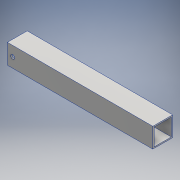
# Autodesk Inventor part: front_arm_rect
Saved by Autodesk Inventor 2016 (Build 200138000, 138)
## iProperties
Created: 2016-09-24
Part Number: front_arm_rect
Material: Aluminum 6061
Document SubType Name: Modeling
Designer: Jakub
Density: 2.7 g/cm^3
Appearance: Aluminum - Flat
Author: Jakub
Autodesk Inventor part; units mm, degrees
ref_plane "YZ Plane" through (0, 0, 0) normal (1, 0, 0) x (0, 1, 0)
ref_plane "XZ Plane" through (0, 0, 0) normal (0, 1, 0) x (-1, 0, 0)
ref_plane "XY Plane" through (0, 0, 0) normal (0, 0, 1) x (1, 0, 0)
sketch "Sketch1" plane through (0, 0, 0) normal (1, 0, 0) x (0, 1, 0)
  line L0 (-7.5, 7.5) -> (7.5, 7.5)
  line L1 (7.5, 7.5) -> (7.5, -7.5)
  line L2 (7.5, -7.5) -> (-7.5, -7.5)
  line L3 (-7.5, -7.5) -> (-7.5, 7.5)
  line L4 (-7.5, 7.5) -> (7.5, -7.5) construction
  line L5 (7.5, 7.5) -> (-7.5, -7.5) construction
  line L6 (-6.5, 6.5) -> (6.5, 6.5)
  line L7 (6.5, 6.5) -> (6.5, -6.5)
  line L8 (6.5, -6.5) -> (-6.5, -6.5)
  line L9 (-6.5, -6.5) -> (-6.5, 6.5)
  line L10 (-6.5, 6.5) -> (6.5, -6.5) construction
  line L11 (6.5, 6.5) -> (-6.5, -6.5) construction
  point P0 (0, 0)
  dimension "d0" = 15
  dimension "d1" = 15
  dimension "d2" = 13
  dimension "d3" = 13
  constraints: 24 end point, 4 midpoint, 4 parallel, 2 horizontal, 2 perpendicular
  measures "d0" distance of L1.end L2.end
  measures "d1" distance of L0.end L1.end
  measures "d2" distance of L7.end L8.end
  measures "d3" distance of L6.end L7.end
extrude "Extrusion1" add sketch "Sketch1" along normal blind 110
sketch "Sketch2" plane through (0, 7.5, 7.5) normal (0, 1, 0) x (1, 0, 0)
  line L0 (0, 7.5) -> (4, 7.5)
  circle A0 centre (4, 7.5) radius 1.5
  dimension "d6" = 4
  dimension "d7" = 3
  constraints: 2 end point, 1 centre point, 1 coincident, 1 horizontal
  measures "d6" distance of L0.start L0.end
  measures "d7" diameter of A0
extrude "Extrusion2" cut sketch "Sketch2" against normal through all
body "Solid1"
